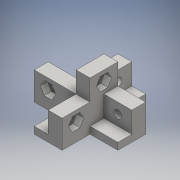
# Autodesk Inventor part: fourwayVer2
Saved by Autodesk Inventor 2016 (Build 200138000, 138)
## iProperties
Created: 2015-11-23
Part Number: fourwayVer2
Material: Generic
Document SubType Name: Modeling
Designer: hesaon
Density: 1 g/cm^3
Appearance: Default
Author: hesaon
Autodesk Inventor part; units mm, degrees
ref_plane "YZ Plane" through (0, 0, 0) normal (1, 0, 0) x (0, 1, 0)
ref_plane "XZ Plane" through (0, 0, 0) normal (0, 1, 0) x (-1, 0, 0)
ref_plane "XY Plane" through (0, 0, 0) normal (0, 0, 1) x (1, 0, 0)
sketch "Sketch1" plane through (0, 0, 0) normal (0, 0, 1) x (1, 0, 0)
  line L0 (0, 0) -> (12, 0)
  line L1 (12, 0) -> (12, 12)
  line L2 (12, 12) -> (0, 12)
  line L3 (0, 12) -> (0, 0)
  line L4 (12, 12) -> (24, 12)
  line L5 (24, 12) -> (24, 0)
  line L6 (24, 0) -> (12, 0)
  line L7 (12, 0) -> (12, 12)
  line L8 (0, 0) -> (-12, 0)
  line L9 (-12, 0) -> (-12, 12)
  line L10 (-12, 12) -> (0, 12)
  line L11 (0, 12) -> (0, 0)
  line L12 (0, 0) -> (12, 0)
  line L13 (12, 0) -> (12, -12)
  line L14 (12, -12) -> (0, -12)
  line L15 (0, -12) -> (0, 0)
  line L16 (0, 12) -> (12, 12)
  line L17 (12, 12) -> (12, 24)
  line L18 (12, 24) -> (0, 24)
  line L19 (0, 24) -> (0, 12)
  dimension "d0" = 12
  dimension "d1" = 12
  dimension "d2" = 12
  dimension "d3" = 12
  dimension "d4" = 12
  dimension "d5" = 12
  dimension "d6" = 12
  dimension "d7" = 12
  dimension "d8" = 12
  dimension "d9" = 12
  constraints: 40 end point, 10 parallel, 5 horizontal, 5 perpendicular
  measures "d0" distance of L2.end L1.end
  measures "d1" distance of L1.end L0.end
  measures "d2" distance of L5.end L6.end
  measures "d3" distance of L4.end L5.end
  measures "d4" distance of L9.end L10.end
  measures "d5" distance of L8.end L9.end
  measures "d6" distance of L13.end L14.end
  measures "d7" distance of L12.end L13.end
  measures "d8" distance of L18.end L17.end
  measures "d9" distance of L17.end L16.end
extrude "Extrusion1" add sketch "Sketch1" along normal blind 12
sketch "Sketch2" plane through (0, 0, 12) normal (0, 0, 1) x (1, 0, 0)
  line L0 (0, 0) -> (0, -12) projected
  line L1 (0, 0) -> (0, 12)
  line L2 (12, 12) -> (12, 24) projected
  line L3 (0, 12) -> (12, 12)
  line L4 (12, -12) -> (12, 0) projected
  line L5 (12, 12) -> (12, 0)
  line L6 (12, 0) -> (0, 0)
  line L7 (0, 6) -> (-12, 6)
  line L8 (-12, 12) -> (-12, 0) projected
  line L9 (12, 6) -> (24, 6)
  line L10 (24, 0) -> (24, 12) projected
  line L11 (6, 12) -> (6, 24)
  line L12 (6, 0) -> (6, -12)
  line L13 (0, -12) -> (12, -12) projected
  line L14 (-12, 6) -> (-12, 12)
  line L15 (0, 12) -> (-12, 12) projected
  line L16 (0, 12) -> (-12, 12)
  line L17 (12, 24) -> (0, 24) projected
  line L18 (6, 24) -> (12, 24)
  line L19 (12, 24) -> (12, 12)
  line L20 (24, 6) -> (24, 0)
  line L21 (6, -12) -> (0, -12)
  line L22 (12, 0) -> (24, 0)
  constraints: 30 end point, 7 midpoint, 5 collinear, 5 perpendicular, 2 vertical
extrude "Extrusion2" cut sketch "Sketch2" against normal blind 9 contours L6 L12 L13 L0 | L7 L8 L15 L1 | L5 L9 L10 L22 | L11 L17 L2 L3
sketch "Sketch3" plane through (6, 12, 12) normal (1, 0, 0) x (0, 0, -1)
  circle A0 centre (4.5, -18) radius 1.725
  line L0 (0, -24) -> (9, -24) projected
  line L1 (9, -24) -> (9, -12) projected
  point P0 (12, -12)
  dimension "d14" = 3.45
  dimension "d15" = 6
  dimension "d16" = 4.5
  constraints: 1 centre point
  measures "d14" diameter of A0
  measures "d15" distance from line of L0 A0.centre
  measures "d16" distance from line of L1 A0.centre
extrude "Extrusion3" cut sketch "Sketch3" along normal blind 3
sketch "Sketch4" plane through (12, -12, 0) normal (1, 0, 0) x (0, 0, -1)
  circle A0 centre (-7.5, 6) radius 1.725 projected
  line L0 (-10.35, 7.6454) -> (-7.5, 9.2909)
  line L1 (-7.5, 9.2909) -> (-4.65, 7.6454)
  line L2 (-4.65, 7.6454) -> (-4.65, 4.3546)
  line L3 (-4.65, 4.3546) -> (-7.5, 2.7091)
  line L4 (-7.5, 2.7091) -> (-10.35, 4.3546)
  line L5 (-10.35, 4.3546) -> (-10.35, 7.6454)
  point P0 (0, 12)
  dimension "d19" = 2.85
  constraints: 12 end point, 1 coincident, 13 other
  measures "d19" distance from line of L5 point (-7.5, 6)
extrude "Extrusion4" cut sketch "Sketch4" against normal blind 3 contours A0 | L0 L1 L2 L3 L4 L5
sketch "Sketch5" plane through (6, 12, 12) normal (1, 0, 0) x (0, 0, -1)
  circle A0 centre (4.5, 6) radius 1.725
  line L0 (12, 12) -> (0, 12) projected
  line L1 (0, 0) -> (0, 12) projected
  point P0 (12, -12)
  dimension "d22" = 3.45
  dimension "d23" = 6
  dimension "d24" = 4.5
  constraints: 1 centre point
  measures "d22" diameter of A0
  measures "d23" distance from line of L0 A0.centre
  measures "d24" distance from line of L1 A0.centre
extrude "Extrusion5" cut sketch "Sketch5" against normal blind 3
sketch "Sketch6" plane through (0, 12, 0) normal (-1, 0, 0) x (0, 0, 1)
  circle A0 centre (7.5, 6) radius 1.725 projected
  line L0 (10.35, 4.3546) -> (7.5, 2.7091)
  line L1 (7.5, 2.7091) -> (4.65, 4.3546)
  line L2 (4.65, 4.3546) -> (4.65, 7.6454)
  line L3 (4.65, 7.6454) -> (7.5, 9.2909)
  line L4 (7.5, 9.2909) -> (10.35, 7.6454)
  line L5 (10.35, 7.6454) -> (10.35, 4.3546)
  point P0 (0, -12)
  dimension "d27" = 2.85
  constraints: 12 end point, 1 coincident, 13 other
  measures "d27" distance from line of L5 point (7.5, 6)
sketch "Sketch7" plane through (0, 0, 12) normal (0, 0, 1) x (1, 0, 0)
  line L0 (6, 12) -> (6, 24) projected
  line L1 (6.0413, 0) -> (6, 0)
  line L2 (6, 0) -> (6, 12)
  line L3 (6, 12) -> (6.0413, 12)
  line L4 (6.0413, 12) -> (6.0413, 0)
  line L5 (12, 0) -> (12, 6) projected
  line L6 (12, 0) -> (12, 12)
  line L7 (24, 12) -> (6, 12) projected
  line L8 (6, 0) -> (12, 0)
  point P0 (0, 0)
  constraints: 12 end point, 2 horizontal, 2 parallel, 1 collinear, 1 perpendicular, 1 point on line
extrude "Extrusion6" add sketch "Sketch7" along normal blind 9 contours L4 L7 L6 L5 L8
extrude "Extrusion7" cut sketch "Sketch6" against normal blind 3 contours A0 | L0 L1 L2 L3 L4 L5
sketch "Sketch8" plane through (12, 12, 0) normal (0, 1, 0) x (1, 0, 0)
  point P0 (-12, 0)
sketch "Sketch9" plane through (12, -12, 0) normal (1, 0, 0) x (0, 0, -1)
  point P0 (0, 12)
sketch "Sketch10" plane through (12, -12, 0) normal (1, 0, 0) x (0, 0, -1)
  point P0 (0, 12)
sketch "Sketch11" plane through (6.0413, 0, 12) normal (-1, 0, 0) x (0, 0, 1)
  circle A0 centre (4.5, 6) radius 1.725
  line L0 (9, 0) -> (0, 0) projected
  line L1 (9, 12) -> (9, 0) projected
  point P0 (-12, 0)
  dimension "d32" = 3.45
  dimension "d33" = 6
  dimension "d34" = 4.5
  constraints: 1 centre point
  measures "d32" diameter of A0
  measures "d33" distance from line of L0 A0.centre
  measures "d34" distance from line of L1 A0.centre
extrude "Extrusion8" cut sketch "Sketch11" against normal blind 3
sketch "Sketch12" plane through (12, -12, 0) normal (1, 0, 0) x (0, 0, -1)
  point P0 (0, 12)
sketch "Sketch13" plane through (12, -12, 0) normal (1, 0, 0) x (0, 0, -1)
  circle A0 centre (-16.5, 18) radius 1.725 projected
  line L0 (-19.35, 19.6454) -> (-16.5, 21.2909)
  line L1 (-16.5, 21.2909) -> (-13.65, 19.6454)
  line L2 (-13.65, 19.6454) -> (-13.65, 16.3546)
  line L3 (-13.65, 16.3546) -> (-16.5, 14.7091)
  line L4 (-16.5, 14.7091) -> (-19.35, 16.3546)
  line L5 (-19.35, 16.3546) -> (-19.35, 19.6454)
  point P0 (0, 12)
  dimension "d37" = 2.85
  constraints: 12 end point, 1 coincident, 13 other
  measures "d37" distance from line of L5 point (-16.5, 18)
extrude "Extrusion9" cut sketch "Sketch13" against normal blind 3 contours A0 | L0 L1 L2 L3 L4 L5
sketch "Sketch14" plane through (12, 6, 12) normal (0, -1, 0) x (1, 0, 0)
  circle A0 centre (6, -4.5) radius 1.725
  line L0 (0, 0) -> (12, 0) projected
  line L1 (12, 0) -> (12, -9) projected
  point P0 (-12, -12)
  dimension "d40" = 3.45
  dimension "d41" = 4.5
  dimension "d42" = 6
  constraints: 1 centre point
  measures "d40" diameter of A0
  measures "d41" distance from line of L0 A0.centre
  measures "d42" distance from line of L1 A0.centre
extrude "Extrusion10" cut sketch "Sketch14" against normal blind 3
sketch "Sketch15" plane through (12, 12, 0) normal (0, 1, 0) x (1, 0, 0)
  circle A0 centre (6, -7.5) radius 1.725 projected
  line L0 (4.3546, -10.35) -> (2.7091, -7.5)
  line L1 (2.7091, -7.5) -> (4.3546, -4.65)
  line L2 (4.3546, -4.65) -> (7.6454, -4.65)
  line L3 (7.6454, -4.65) -> (9.2909, -7.5)
  line L4 (9.2909, -7.5) -> (7.6454, -10.35)
  line L5 (7.6454, -10.35) -> (4.3546, -10.35)
  point P0 (-12, 0)
  dimension "d45" = 2.85
  constraints: 12 end point, 1 coincident, 13 other
  measures "d45" distance from line of L5 point (6, -7.5)
extrude "Extrusion11" cut sketch "Sketch15" against normal blind 3 contours A0 | L0 L1 L2 L3 L4 L5
sketch "Sketch16" plane through (-12, 6, 12) normal (0, 1, 0) x (1, 0, 0)
  circle A0 centre (6, 4.5) radius 1.725
  line L0 (12, 0) -> (0, 0) projected
  line L1 (0, 0) -> (0, 9) projected
  point P0 (12, 12)
  dimension "d48" = 3.45
  dimension "d49" = 4.5
  dimension "d50" = 6
  constraints: 1 centre point
  measures "d48" diameter of A0
  measures "d49" distance from line of L0 A0.centre
  measures "d50" distance from line of L1 A0.centre
extrude "Extrusion12" cut sketch "Sketch16" against normal blind 3
sketch "Sketch17" plane through (-12, 0, 0) normal (0, -1, 0) x (1, 0, 0)
  circle A0 centre (6, 7.5) radius 1.725 projected
  line L0 (4.3546, 4.65) -> (2.7091, 7.5)
  line L1 (2.7091, 7.5) -> (4.3546, 10.35)
  line L2 (4.3546, 10.35) -> (7.6454, 10.35)
  line L3 (7.6454, 10.35) -> (9.2909, 7.5)
  line L4 (9.2909, 7.5) -> (7.6454, 4.65)
  line L5 (7.6454, 4.65) -> (4.3546, 4.65)
  point P0 (12, 0)
  dimension "d53" = 2.85
  constraints: 12 end point, 1 coincident, 13 other
  measures "d53" distance from line of L2 point (6, 7.5)
extrude "Extrusion13" cut sketch "Sketch17" against normal blind 3 contours A0 | L0 L1 L2 L3 L4 L5
body "Solid1"
